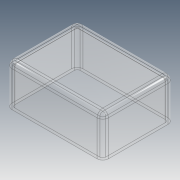
# Autodesk Inventor part: Fuse Box 6-way-lid
Saved by Autodesk Inventor 2020 (Build 240168000, 168)
## iProperties
Created: 2021-05-31
Part Number: Fuse Box 6-way-lid
Material: PMMA Plastic
Document SubType Name: Modeling
Designer: Simon.Alvarez
Density: 1.188 g/cm^3
Appearance: Polycarbonate - Clear
Author: Simon.Alvarez
Autodesk Inventor part; units mm, degrees
ref_plane "YZ Plane" through (0, 0, 0) normal (1, 0, 0) x (0, 1, 0)
ref_plane "XZ Plane" through (0, 0, 0) normal (0, 1, 0) x (-1, 0, 0)
ref_plane "XY Plane" through (0, 0, 0) normal (0, 0, 1) x (1, 0, 0)
sketch "Sketch1" plane through (0, 0, 0) normal (0, 1, 0) x (-1, 0, 0)
  line L0 (30, 25) -> (-30, 25)
  line L1 (-34, 21) -> (-34, -21)
  line L2 (-30, -25) -> (30, -25)
  line L3 (34, -21) -> (34, 21)
  line L4 (34, 25) -> (-34, -25) construction
  line L5 (-34, 25) -> (34, -25) construction
  arc A0 (30, -25) -> (34, -21) centre (30, -21) ccw
  arc A1 (34, 21) -> (30, 25) centre (30, 21) ccw
  arc A2 (-30, 25) -> (-34, 21) centre (-30, 21) ccw
  arc A3 (-34, -21) -> (-30, -25) centre (-30, -21) ccw
  point P0 (0, 0)
  dimension "d0" = 68
  dimension "d1" = 50
  dimension "d2" = 4
  constraints: 12 end point, 8 point on circle, 8 point on line, 8 tangent, 4 centre point, 3 equal radius, 2 midpoint, 2 parallel, 1 horizontal, 1 perpendicular
  measures "d0" distance of L4.end L5.end
  measures "d1" distance of L5.end L4.start
  measures "d2" radius of A0
extrude "Extrusion1" add sketch "Sketch1" along normal blind 29
fillet "Fillet1" radius 4 8 edges at (32.8284, 29, 23.8284) (34, 29, 0) (32.8284, 29, -23.8284) (0, 29, -25) (-32.8284, 29, -23.8284) (-34, 29, 0) (-32.8284, 29, 23.8284) (0, 29, 25)
shell "Shell1" thickness 2 removed faces 1 at (10, 0, 8.3333)
body "Solid1"
